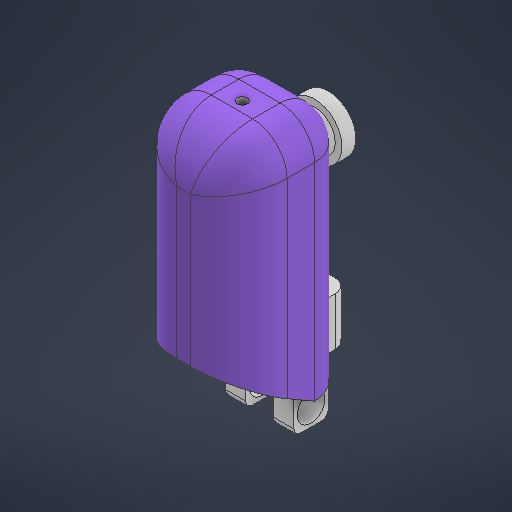
# Autodesk Inventor part: Part1
Saved by Autodesk Inventor 2026 (Build 300175050, 175E)
## iProperties
Created: 2026-05-22
Part Number: Part1
Material: Generic
Document SubType Name: Modeling
Designer: SaiAn
Density: 1 g/cm^3
Appearance: Default
Author: SaiAn
Autodesk Inventor part; units mm, degrees
ref_plane "YZ Plane" through (0, 0, 0) normal (1, 0, 0) x (0, 1, 0)
ref_plane "XZ Plane" through (0, 0, 0) normal (0, 1, 0) x (-1, 0, 0)
ref_plane "XY Plane" through (0, 0, 0) normal (0, 0, 1) x (1, 0, 0)
sketch "Sketch1" plane through (0, 0, 0) normal (0, 0, 1) x (1, 0, 0)
  line L0 (0, 0) -> (16, 0)
  line L1 (16, 0) -> (16, 30)
  line L2 (11, 35) -> (5, 35)
  line L3 (0, 30) -> (0, 0)
  arc A0 (16, 30) -> (11, 35) centre (11, 30) ccw
  arc A1 (5, 35) -> (0, 30) centre (5, 30) ccw
  point P0 (16, 35)
  point P1 (0, 35)
  dimension "d0" = 16
  dimension "d1" = 35
  dimension "d2" = 5
  constraints: 8 end point, 4 point on circle, 4 point on line, 4 tangent, 2 centre point, 2 parallel, 1 equal radius, 1 horizontal, 1 perpendicular
  measures "d0" distance of point (0, 35) point (16, 35)
  measures "d1" distance of point (16, 35) L0.end
  measures "d2" radius of A0
extrude "Extrusion1" add sketch "Sketch1" along normal blind 16
fillet "Fillet1" radius 5 5 edges at (8, 35, 0) (1.4645, 33.5355, 0) (0, 15, 0) (16, 15, 0) (14.5355, 33.5355, 0)
sketch "Sketch2" plane through (16, 0, 16) normal (1, 0, 0) x (0, 0, -1)
  line L0 (11, 0) -> (0, 0) projected
  line L1 (11, 0) -> (0, 6.3509)
  line L2 (0, 0) -> (0, 30) projected
  line L3 (11, 0) -> (23.7017, 0) construction
  line L4 (0, 6.3509) -> (0, 0)
  line L5 (0, 0) -> (11, 0)
  point P0 (16, 0)
  dimension "d6" = 150
  constraints: 8 end point, 1 equal length, 1 horizontal, 1 perpendicular, 1 point on line, 1 vertical
  measures "d6" angle of L3 L1
extrude "Extrusion2" cut sketch "Sketch2" against normal through all
fillet "Fillet2" radius 7 5 edges at (8, 35, 16) (1.4645, 33.5355, 16) (0, 18.1754, 16) (16, 18.1754, 16) (14.5355, 33.5355, 16)
sketch "Sketch3" plane through (5, 0, 0) normal (0, -1, 0) x (1, 0, 0)
  line L0 (11, 9) -> (11, 5) projected
  line L1 (-5, 5) -> (-5, 9) projected
  line L2 (6, 0) -> (0, 0) projected
  line L3 (11, 5) -> (-5, 5) projected
  line L4 (5, 0) -> (8, 0)
  line L5 (8, 0) -> (8, 5)
  line L6 (8, 5) -> (5, 5)
  line L7 (5, 5) -> (5, 0)
  line L8 (2, 0) -> (-2, 0)
  line L9 (-2, 0) -> (-2, 5)
  line L10 (-2, 5) -> (1, 5)
  line L11 (1, 5) -> (1, 0)
  point P0 (-5, 0)
  point P1 (3, 2.5)
  point P2 (2, 5)
  point P3 (5, 0)
  point P4 (-2, 5)
  point P5 (1, 0)
  point P6 (1, 5)
  dimension "d53" = 3
  dimension "d54" = 3
  dimension "d59" = 3
  dimension "d60" = 3
  dimension "d61" = 5
  constraints: 16 end point, 4 point on line, 3 parallel, 3 perpendicular, 2 horizontal
  measures "d53" distance of L6.end L5.end
  measures "d54" distance of L9.end L10.end
  measures "d59" distance from line of L0.end L5
  measures "d60" distance from line of L1.start L9
  measures "d61" distance of L4.end L5.end
extrude "Extrusion3" add sketch "Sketch3" along normal blind 6 contours L2 L7 L3 L5 L4 | L2 L8 L9 L3 L11
sketch "Sketch5" plane through (0, 0, 0) normal (0, 0, -1) x (-1, 0, 0)
  circle A0 centre (-8, 26) radius 3
  line L0 (-5, 30) -> (-5, 0) projected
  point P0 (0, 0)
  constraints: 1 centre point, 1 tangent
extrude "Extrusion5" add sketch "Sketch5" along normal blind 5
sketch "Sketch6" plane through (8, 26, -5) normal (0, 0, -1) x (-1, 0, 0)
  circle A0 centre (0, 0) radius 4
  point P0 (8, -26)
  dimension "d24" = 8
  constraints: 1 centre point
  measures "d24" diameter of A0
extrude "Extrusion6" add sketch "Sketch6" against normal blind 2
sketch "Sketch9" plane through (0, 0, 0) normal (0, 0, -1) x (-1, 0, 0)
  line L0 (-5, 0) -> (-11, 0) projected
  line L1 (-11, 0) -> (-9, 0)
  line L2 (-9, 0) -> (-9, 7)
  line L3 (-9, 7) -> (-11, 7)
  line L4 (-11, 7) -> (-11, 0)
  line L5 (-5, 0) -> (-7, 0)
  line L6 (-7, 0) -> (-7, 7)
  line L7 (-7, 7) -> (-5, 7)
  line L8 (-5, 7) -> (-5, 0)
  point P0 (0, 0)
  dimension "d35" = 2
  dimension "d36" = 7
  dimension "d37" = 2
  dimension "d38" = 7
  constraints: 16 end point, 4 parallel, 2 horizontal, 2 perpendicular
  measures "d35" distance of L3.end L2.end
  measures "d36" distance of L2.end L1.end
  measures "d37" distance of L6.end L7.end
  measures "d38" distance of L5.end L6.end
extrude "Extrusion9" add sketch "Sketch9" along normal blind 3
sketch "Sketch10" plane through (0, 0, -3) normal (0, 0, -1) x (-1, 0, 0)
  line L0 (-11, 7) -> (-9, 7) projected
  line L1 (-5, 7) -> (-5, 0) projected
  line L2 (-11, 7) -> (-5, 7)
  line L3 (-5, 7) -> (-5, 0)
  line L4 (-5, 0) -> (-11, 0)
  line L5 (-11, 0) -> (-11, 7)
  point P0 (0, 0)
  dimension "d41" = 6
  dimension "d42" = 7
  constraints: 8 end point, 2 parallel, 1 horizontal, 1 perpendicular
  measures "d41" distance of L1.end L4.end
  measures "d42" distance of L2.end L1.end
extrude "Extrusion10" add sketch "Sketch10" along normal blind 2
sketch "Sketch11" plane through (0, 0, 5) normal (0, -1, 0) x (1, 0, 0)
  circle A0 centre (8, 2.5) radius 0.75
  point P0 (0, -5)
  dimension "d45" = 1.5
  constraints: 1 centre point
  measures "d45" diameter of A0
extrude "Extrusion11" cut sketch "Sketch11" against normal through all
fillet "Fillet4" radius 2 2 edges at (11, 3.5, -5) (5, 3.5, -5)
sketch "Sketch12" plane through (0, 0, 5) normal (0, -1, 0) x (1, 0, 0)
  circle A0 centre (8, -6.5) radius 0.75
  point P0 (0, -5)
  dimension "d49" = 1.5
  constraints: 1 centre point
  measures "d49" diameter of A0
extrude "Extrusion12" cut sketch "Sketch12" against normal through all
sketch "Sketch13" plane through (3, 0, 0) normal (-1, 0, 0) x (0, 0, 1)
  circle A0 centre (2.5, -3.5) radius 2.025
  point P0 (0, 0)
  dimension "d55" = 4.05
  constraints: 1 centre point
  measures "d55" diameter of A0
extrude "Extrusion13" cut sketch "Sketch13" against normal through all
fillet "Fillet5" radius 1 4 edges at (4.5, -6, 0) (11.5, -6, 0) (4.5, -6, 5) (11.5, -6, 5)
body "Solid1"
